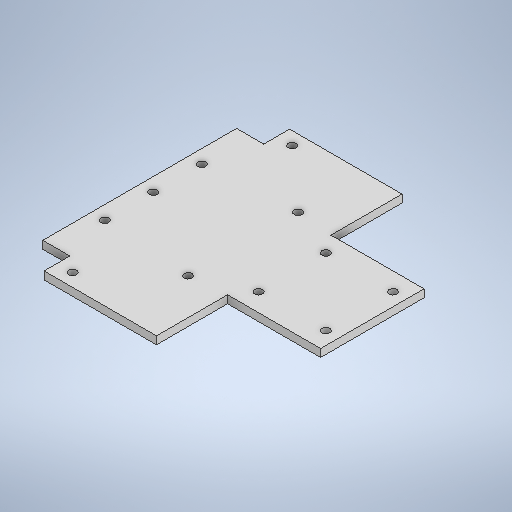
# Autodesk Inventor part: basePlate
Saved by Autodesk Inventor 2025.1 (Build 291241020, 241B)
## iProperties
Created: 2025-04-15
Part Number: basePlate
Material: Generic
Document SubType Name: Modeling
Designer: omiye
Density: 1 g/cm^3
Appearance: Default
Author: omiye
Autodesk Inventor part; units mm, degrees
ref_plane "YZ Plane" through (0, 0, 0) normal (1, 0, 0) x (0, 1, 0)
ref_plane "XZ Plane" through (0, 0, 0) normal (0, 1, 0) x (-1, 0, 0)
ref_plane "XY Plane" through (0, 0, 0) normal (0, 0, 1) x (1, 0, 0)
sketch "Sketch1" plane through (0, 0, 0) normal (0, 1, 0) x (-1, 0, 0)
  line L0 (-45, 0) -> (-45, 6)
  line L1 (-45, 6) -> (-45, -6)
  line L2 (-45, 6) -> (-45, 20)
  line L3 (-45, 20) -> (-45, -6)
  line L4 (-45, -6) -> (-45, -20)
  line L5 (-45, 20) -> (-9, 20)
  line L6 (-45, -20) -> (-9, -20)
  line L7 (-45, -20) -> (-9, -20)
  line L8 (-9, 20) -> (-9, 47.5)
  line L9 (-45, 6) -> (-45, 20)
  circle A0 centre (-14, 13) radius 1.55
  circle A1 centre (-14, -13) radius 1.55
  circle A2 centre (-40, 13) radius 1.55
  circle A3 centre (-40, -13) radius 1.55
  line L10 (-45, 20) -> (-45, -20)
  line L11 (-9, 20) -> (-45, 20)
  line L12 (-45, 20) -> (-45, -20)
  line L13 (-45, -20) -> (-9, -20)
  line L14 (45, 37.5) -> (34.5, 37.5)
  line L15 (45, -37.5) -> (34.5, -37.5)
  line L16 (34.5, -37.5) -> (34.5, -47.5)
  line L17 (34.5, 37.5) -> (34.5, 47.5)
  circle A4 centre (28.5, 42.5) radius 1.55
  circle A5 centre (28.5, -42.5) radius 1.55
  line L18 (34.5, -47.5) -> (-5, -47.5)
  line L19 (45, -37.5) -> (45, 37.5)
  line L20 (34.5, 47.5) -> (-9, 47.5)
  line L21 (-9, -20) -> (-9, -47.5)
  line L22 (-9, -47.5) -> (-5, -47.5)
  circle A6 centre (5, 21.3) radius 1.55
  circle A7 centre (5, -21.3) radius 1.55
  circle A8 centre (39.75, 18.75) radius 1.55
  circle A9 centre (39.75, 0) radius 1.55
  circle A10 centre (39.75, -18.75) radius 1.55
  point P0 (0, 0)
  dimension "d2" = 6
  dimension "d3" = 12
  dimension "d4" = 14
  dimension "d5" = 14
  dimension "d6" = 36
  dimension "d7" = 36
  dimension "d13" = 3.1
  dimension "d14" = 3.1
  dimension "d15" = 3.1
  dimension "d17" = 10.5
  dimension "d19" = 10.5
  dimension "d22" = 3.1
  dimension "d23" = 3.1
  dimension "d27" = 3.1
  dimension "d28" = 3.1
  dimension "d32" = 3.1
  dimension "d33" = 3.1
  dimension "d34" = 3.1
  constraints: 46 end point, 11 centre point, 4 perpendicular, 3 collinear, 1 horizontal, 1 point on line, 1 vertical
  measures "d2" distance of L0.start L0.end
  measures "d3" distance of L0.end L1.end
  measures "d4" distance of L0.end L2.end
  measures "d5" distance of L1.end L4.end
  measures "d6" distance of L2.end L5.end
  measures "d7" distance of L4.end L6.end
  measures "d13" diameter of A0
  measures "d14" diameter of A1
  measures "d15" diameter of A3
  measures "d17" distance of L14.start L14.end
  measures "d19" distance of L15.start L15.end
  measures "d22" diameter of A4
  measures "d23" diameter of A5
  measures "d27" diameter of A6
  measures "d28" diameter of A7
  measures "d32" diameter of A8
  measures "d33" diameter of A9
  measures "d34" diameter of A10
extrude "Extrusion2" add sketch "Sketch1" along normal blind 3
body "Solid2"
